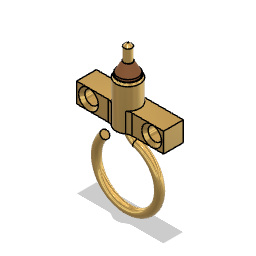
electrode puck v2 connector v8 (Autodesk Fusion 360 design; units mm, degrees)
Autodesk Fusion 360 part; units mm, degrees
note: some values were not read from the file. Set by a fixed rule: which sketch regions a step uses.
sketch "Sketch1" plane through (0, 0, 0) normal (0, 1, 0) x (1, 0, 0)
  circle A0 centre (0, 0) radius 0.5
  circle A1 centre (0, 0) radius 1.25
  circle A2 centre (0, 0) radius 1.5
  line L0 (-5.5, 1.5) -> (5.5, 1.5)
  line L1 (5.5, 1.5) -> (5.5, -1)
  line L2 (5.5, -1) -> (1.118, -1)
  line L3 (-1.118, -1) -> (-5.5, -1)
  line L4 (-5.5, -1) -> (-5.5, 1.5)
  line L5 (0, -20) -> (0, -2.5) construction
  dimension "d1" = 1
  dimension "d2" = 2.5
  dimension "d3" = 3
  dimension "d4" = 2.5
  dimension "d17" = 11
  constraint coincident A0.centre A1.centre
  constraint horizontal L0
  constraint perpendicular L0 L1
  constraint perpendicular L1 L2
  constraint perpendicular L0 L4
  constraint perpendicular L3 L4
  constraint tangent A2 L0
  constraint collinear L2 L3
  constraint coincident A2 L2.end
  constraint coincident A2 L3.start
  measures "d1" diameter of A0
  measures "d2" diameter of A1
  measures "d3" diameter of A2
  measures "d4" distance of L0.end L1.end
  measures "d17" distance of L1 L4
extrude "Extrude1" add sketch "Sketch1" along normal blind 2.5 contours A2 | A2 L0 L3 L4 | A2 L0 L1 L2 makes body 1
extrude "Extrude2" add sketch "Sketch1" along normal blind 5.5 contours A2 bodies 1
fillet "Fillet1" radius 1 2 edges at (1.118, 1.25, 1) (-1.118, 1.25, 1) on bodies 1
extrude "Extrude3" add sketch "Sketch1" along normal blind 7 separate body contours A1 makes body 2
extrude "Extrude4" add sketch "Sketch1" along normal blind 9 separate body contours A0 makes body 3
chamfer "Chamfer1" distance 0.4 angle 45 1 edges at (-0.4662, 9, 0.1808) on bodies 3
sketch "Sketch2" plane through (0, 0, 0) normal (0, 0, 1) x (1, 0, 0)
  arc A0 (0, 0) -> (1.0909, -1.4431) centre (1.5, 0) ccw
  arc A1 (-2.927, -2.5652) -> (1.0909, -1.4431) centre (0, -5.2915) ccw
  dimension "d19" = 1.5
  dimension "d20" = 4
  constraint tangent A0 A1
  constraint coincident A0.start origin
  constraint horizontal A0.centre A0.start
  constraint vertical A1.centre A0.start
  measures "d19" radius of A0
  measures "d20" radius of A1
sweep "Sweep1" add profiles "Sketch1" path "Sketch2" along A0 A1 section 1 contours A0 bodies 3
sketch "Sketch3" plane through (0, 0, 1) normal (0, 0, 1) x (-1, 0, 0)
  line L0 (-5.5, 0) -> (5.5, 0)
  line L1 (0, 1.75) -> (0, 22.5) construction
  line L2 (-5.5, -1.25) -> (5.5, -1.25) construction
  line L3 (-1.5, -2.5) -> (-1.5, 0)
  line L4 (-1.5, 0) -> (-5.5, 0)
  line L5 (-5.5, 0) -> (-5.5, -2.5)
  line L6 (-5.5, -2.5) -> (-1.5, -2.5)
  point P0 (-4, -1.25)
  point P1 (4, -1.25)
  dimension "d27" = 8
  constraint symmetric P0 P1 L1
  constraint coincident P0 L2
  constraint midpoint L2.start L5
  constraint horizontal L2
  measures "d27" distance of P0 P1
hole "Hole1" at (4, 1.25, 1) at (-4, 1.25, 1) direction (0, 0, -1) diameter 1.7 depth 6 tip angle 118 countersink diameter 2.5 countersink angle 90 bodies 1
chamfer "Chamfer2" distance 0.7 angle 60 1 edges at (-1.1654, 7, 0.452) measured on face at (0.9935, 7, 0.0869) on bodies 2
chamfer "Chamfer3" distance 0.15 angle 65 1 edges at (-1.3985, 5.5, 0.5424) measured on face at (-1.3264, 5.5, 0.4871) on bodies 1
copy_body "Body->Comp1" bodies 1 removing the originals makes body 4 in component "main gnd"
copy_body "Body->Comp2" bodies 2 removing the originals makes body 5 in component "dielectric"
copy_body "Body->Comp3" bodies 3 removing the originals makes body 6 in component "conductor"
component "main gnd" placed x (1, 0, 0) y (0, 1, 0) z (0, 0, 1) at (0, 0, 0)
component "dielectric" placed x (1, 0, 0) y (0, 1, 0) z (0, 0, 1) at (0, 0, 0)
component "conductor" placed x (1, 0, 0) y (0, 1, 0) z (0, 0, 1) at (0, 0, 0)
named bodies: "main gnd", "dielectric", "conductor"
